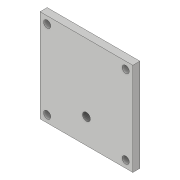
# Autodesk Inventor part: 2
Saved by Autodesk Inventor 2019 (Build 230136000, 136)
## iProperties
Created: 2019-10-07
Part Number: 2
Material: Generic
Document SubType Name: Modeling
Designer: Admin
Density: 1 g/cm^3
Appearance: Default
Author: Admin
Autodesk Inventor part; units mm, degrees
ref_plane "YZ Plane" through (0, 0, 0) normal (1, 0, 0) x (0, 1, 0)
ref_plane "XZ Plane" through (0, 0, 0) normal (0, 1, 0) x (-1, 0, 0)
ref_plane "XY Plane" through (0, 0, 0) normal (0, 0, 1) x (1, 0, 0)
sketch "Sketch1" plane through (0, 0, 0) normal (0, 0, 1) x (1, 0, 0)
  line L0 (0, 0) -> (130, 0)
  line L1 (130, 0) -> (130, 130)
  line L2 (130, 130) -> (0, 130)
  line L3 (0, 130) -> (0, 0)
  dimension "d0" = 130
  dimension "d1" = 130
  constraints: 8 end point, 2 parallel, 1 horizontal, 1 perpendicular
  measures "d0" distance of L2.end L1.end
  measures "d1" distance of L1.end L0.end
extrude "Extrusion1" add sketch "Sketch1" along normal blind 10
sketch "Sketch2" plane through (0, 0, 10) normal (0, 0, 1) x (1, 0, 0)
  line L0 (130, 130) -> (0, 130) projected
  line L1 (0, 130) -> (10, 130)
  line L2 (10, 130) -> (10, 0)
  line L3 (10, 0) -> (120, 0)
  line L4 (0, 0) -> (130, 0) projected
  line L5 (120, 0) -> (120, 130)
  line L6 (120, 130) -> (120, 120)
  line L7 (120, 120) -> (10, 120)
  line L8 (130, 0) -> (130, 10)
  line L9 (130, 0) -> (130, 130) projected
  line L10 (130, 10) -> (0, 10)
  line L11 (0, 130) -> (0, 0) projected
  circle A0 centre (10, 120) radius 5
  circle A1 centre (120, 120) radius 5
  circle A2 centre (120, 10) radius 5
  circle A3 centre (10, 10) radius 5
  dimension "d4" = 10
  dimension "d5" = 130
  dimension "d6" = 110
  dimension "d7" = 10
  dimension "d8" = 10
  dimension "d9" = 130
  dimension "d10" = 10
  dimension "d11" = 10
  dimension "d12" = 10
  dimension "d13" = 10
  constraints: 16 end point, 11 point on line, 4 centre point, 2 coincident, 2 perpendicular
  measures "d4" distance of L0.end L1.end
  measures "d5" distance of L1.end L2.end
  measures "d6" distance of L2.end L3.end
  measures "d7" distance of L5.end L6.end
  measures "d8" distance of L4.end L8.end
  measures "d9" distance of L8.end L10.end
  measures "d10" diameter of A0
  measures "d11" diameter of A1
  measures "d12" diameter of A2
  measures "d13" diameter of A3
extrude "Extrusion2" cut sketch "Sketch2" against normal through all contours A1 L5 | L5 L7 A1 | A2 L5 L10 | L10 L5 A2 | A0 L7 L2 | L2 A0 | L5 A1 L7 | L10 A2 L5 | L5 A2 L10 | L7 A0 L2 | A3 L2 L10 | L10 L2 A3 | A3 L10 L2 | L2 L10 A3
sketch "Sketch3" plane through (0, 0, 10) normal (0, 0, 1) x (1, 0, 0)
  line L0 (0, 0) -> (130, 0) projected
  line L1 (65, 0) -> (30, 0)
  line L2 (65, 0) -> (65, 35)
  circle A0 centre (65, 35) radius 5.5
  dimension "d16" = 65
  dimension "d17" = 35
  dimension "d18" = 35
  dimension "d19" = 11
  constraints: 4 end point, 1 centre point, 1 coincident, 1 midpoint, 1 vertical
  measures "d16" distance of L0.start L1.start
  measures "d17" distance of L1.start L1.end
  measures "d18" distance of L1.start L2.end
  measures "d19" diameter of A0
extrude "Extrusion3" cut sketch "Sketch3" against normal through all
thread "Thread1" size "M11x1.5" class "6H" standard "ANSI Metric M Profile" full length
body "Solid1"
